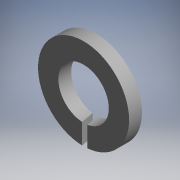
# Autodesk Inventor part: SPRING_WASHER5.1-9.2-1.3
Saved by Autodesk Inventor 2017.3 (Build 213256000, 256)
## iProperties
Part Number: SPRING_WASHER5.1-9.2-1.3
Material: Generic
Catalog Web Link: www.cadenas.de
Description: SPRING_WASHER-Spring_Washer
Vendor: MISUMI
Document SubType Name: Modeling
Designer: partserver
Manufacturer: MISUMI
Mass: 0.0584806 g
Surface Area: 1.52452 cm^2
Volume: 0.0584806 cm^3
Density: 1 g/cm^3
Appearance: PSOLRGB-192-192-192
Category: PARTsolutions
Company: MISUMI
Title: SPRING_WASHER5.1-9.2-1.3
Author: Cadenas PARTsolutions
Comments: Spring_Washer
PSOL_IDENT_0: {$CADENAS_DATA\23d-libs\misumi\metric\accessories\spring_washer.prj},209 {VTYP=3D},{NB=SPRING_WASHER
PSOL_IDENT_1: 5.1-9.2-1.3},{LINA=SPRING_WASHER5.1-9.2-1.3},{NN=SPRING_WASHER},{DATE=12.12.2019 00:48:26},{GEOMDATE=
PSOL_IDENT_2: 28.02.2014 02:17:00},{VERSION=},{LINEID=10},{WBVAR=DD,D,TT},{WBNUMERIC=DD,D,TT}  {NB=SPRING_WASHER5.
PSOL_IDENT_3: 1-9.2-1.3},{LINA=SPRING_WASHER5.1-9.2-1.3},{KT=DUMMY},{PN=SPRING_WASHER5.1-9.2-1.3},{TYPE=SPRING_WAS
PSOL_IDENT_4: HER},{DD=5.1},{DMIN=6.1},{D=9.2},{TT=1.3}
NB: SPRING_WASHER5.1-9.2-1.3
NN: SPRING_WASHER
NT: Spring_Washer
NBSYN: $PN.
LINA: SPRING_WASHER5.1-9.2-1.3
CATALOG: Misumi
PN: SPRING_WASHER5.1-9.2-1.3
TYPE: SPRING_WASHER
DD: 5.1
D: 9.2
TT: 1.3
SUPPLIER: MISUMI
ARTICLENO: SPRING_WASHER5.1-9.2-1.3
BOMINFO: SPRING_WASHER5.1-9.2-1.3
CREATOR: CADENAS GmbH
Autodesk Inventor part; units mm, degrees
ref_plane "YZ Plane" through (0, 0, 0) normal (1, 0, 0) x (0, 1, 0)
ref_plane "XZ Plane" through (0, 0, 0) normal (0, 1, 0) x (-1, 0, 0)
ref_plane "XY Plane" through (0, 0, 0) normal (0, 0, 1) x (1, 0, 0)
sketch "Sketch_1" plane through (0, 0, 0) normal (0, 0, 1) x (1, 0, 0)
  line L0 (0, -50) -> (0, 50)
  line L1 (2.55, -0.65) -> (4.6, -0.65)
  line L2 (4.6, -0.65) -> (4.6, 0.65)
  line L3 (4.6, 0.65) -> (2.55, 0.65)
  line L4 (2.55, 0.65) -> (2.55, -0.65)
  constraints: 10 end point
revolve "Revolution1" add sketch "Sketch_1" angle 360 about axis through (0, -50, 0) along (0, -1, 0)
sketch "Sketch_3" plane through (0, 0, 0) normal (0, 0, 1) x (1, 0, 0)
  line L0 (-0.4769, -1.236) -> (0.0254, -1.3245)
  line L1 (0.0254, -1.3245) -> (0.4769, 1.236)
  line L2 (0.4769, 1.236) -> (-0.0254, 1.3245)
  line L3 (-0.0254, 1.3245) -> (-0.4769, -1.236)
  constraints: 8 end point
extrude "Extrusion1" cut sketch "Sketch_3" along normal blind 5.6
ref_plane "CP_XY" through (0, -0.65, 0) normal (0, -1, 0) x (1, 0, 0)
ref_plane "CP_YZ" through (0, -0.65, 0) normal (1, 0, 0) x (0, 0, 1)
ref_plane "CP_ZX" through (0, -0.65, 0) normal (0, 0, 1) x (0, -1, 0)
ref_plane "to_bolt_XY" through (0, 0.65, 0) normal (0, 1, 0) x (1, 0, 0)
ref_plane "to_bolt_YZ" through (0, 0.65, 0) normal (1, 0, 0) x (0, 0, -1)
ref_plane "to_bolt_ZX" through (0, 0.65, 0) normal (0, 0, -1) x (0, 1, 0)
body "Solid1"
